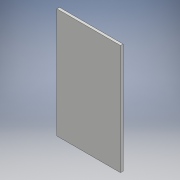
# Autodesk Inventor part: RaspberryPi
Saved by Autodesk Inventor 2018 (Build 220112000, 112)
## iProperties
Created: 2017-10-07
Part Number: RaspberryPi
Material: Generic
Document SubType Name: Modeling
Designer: Akram Al-Hourani
Density: 1 g/cm^3
Appearance: Default
Author: Akram Al-Hourani
Autodesk Inventor part; units mm, degrees
ref_plane "YZ Plane" through (0, 0, 0) normal (1, 0, 0) x (0, 1, 0)
ref_plane "XZ Plane" through (0, 0, 0) normal (0, 1, 0) x (-1, 0, 0)
ref_plane "XY Plane" through (0, 0, 0) normal (0, 0, 1) x (1, 0, 0)
sketch "Sketch1" plane through (0, 0, 0) normal (0, 1, 0) x (-1, 0, 0)
  line L0 (-24.5, 42.5) -> (24.5, 42.5)
  line L1 (24.5, 42.5) -> (24.5, -42.5)
  line L2 (24.5, -42.5) -> (-24.5, -42.5)
  line L3 (-24.5, -42.5) -> (-24.5, 42.5)
  line L4 (-24.5, 42.5) -> (24.5, -42.5) construction
  line L5 (24.5, 42.5) -> (-24.5, -42.5) construction
  point P0 (0, 0)
  dimension "d0" = 49
  dimension "d1" = 85
  constraints: 12 end point, 2 midpoint, 2 parallel, 1 horizontal, 1 perpendicular
  measures "d0" distance of L1.end L2.end
  measures "d1" distance of L0.end L1.end
extrude "Extrusion1" add sketch "Sketch1" along normal blind 2
body "Solid1"
